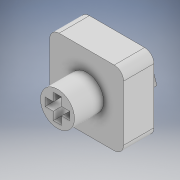
# Autodesk Inventor part: IPC A-CAL 9 key
Saved by Autodesk Inventor 2022 (Build 260153000, 153)
## iProperties
Created: 2021-12-31
Part Number: IPC A-CAL 9 key
Material: Generic
Document SubType Name: Modeling
Designer: solor
Density: 1 g/cm^3
Appearance: Default
Author: solor
Autodesk Inventor part; units mm, degrees
ref_plane "YZ Plane" through (0, 0, 0) normal (1, 0, 0) x (0, 1, 0)
ref_plane "XZ Plane" through (0, 0, 0) normal (0, 1, 0) x (-1, 0, 0)
sketch "Sketch1" plane through (0, 0, 0) normal (0, 0, 1) x (1, 0, 0)
  line L0 (14.6962, 12.74) -> (14.6962, 0) construction
  line L1 (10.61, 12.2) -> (1.53, 12.2)
  arc A0 (1.53, 12.2) -> (0, 10.67) centre (1.53, 10.67) ccw
  line L2 (0, 10.67) -> (0, 1.53)
  arc A1 (0, 1.53) -> (1.53, 0) centre (1.53, 1.53) ccw
  line L3 (1.53, 0) -> (10.61, 0)
  arc A2 (10.61, 0) -> (12.14, 1.53) centre (10.61, 1.53) ccw
  arc A3 (12.14, 10.67) -> (10.61, 12.2) centre (10.61, 10.67) ccw
  line L4 (12.14, 10.67) -> (12.14, 1.53)
  point P0 (0, 0)
  point P1 (0, 0)
  dimension "d10" = 12.74
  constraints: 10 end point, 8 point on circle, 4 centre point, 2 vertical, 1 point on line
  measures "d10" distance of L0.start L0.end
ref_plane "Work Plane1" through (0, 0, 5) normal (0, 0, 1) x (1, 0, 0)
sketch "Sketch2" plane through (0, 0, 5) normal (0, 0, 1) x (1, 0, 0)
  line L0 (10.88, 12.74) -> (1.8, 12.74) projected
  line L1 (10.88, 12.74) -> (1.8, 12.74) projected
  arc A0 (1.8, 12.74) -> (0, 10.94) centre (1.8, 10.94) ccw projected
  line L2 (0, 10.94) -> (0, 1.8) projected
  arc A1 (0, 1.8) -> (1.8, 0) centre (1.8, 1.8) ccw projected
  line L3 (1.8, 0) -> (10.88, 0) projected
  arc A2 (10.88, 0) -> (12.68, 1.8) centre (10.88, 1.8) ccw projected
  line L4 (12.68, 1.8) -> (12.68, 10.94) projected
  arc A3 (12.68, 10.94) -> (10.88, 12.74) centre (10.88, 10.94) ccw projected
  circle A4 centre (6.34, 6.37) radius 2.8
  line L5 (5.665, 8.395) -> (7.015, 8.395)
  line L6 (7.015, 4.345) -> (5.665, 4.345)
  line L7 (5.665, 4.345) -> (7.015, 8.395) construction
  line L8 (5.665, 8.395) -> (7.015, 4.345) construction
  line L9 (8.365, 5.695) -> (8.365, 7.045)
  line L10 (4.315, 7.045) -> (4.315, 5.695)
  line L11 (4.315, 5.695) -> (8.365, 7.045) construction
  line L12 (8.365, 5.695) -> (4.315, 7.045) construction
  line L13 (4.315, 5.695) -> (5.665, 5.695)
  line L14 (7.015, 5.695) -> (8.365, 5.695)
  line L15 (5.665, 4.345) -> (5.665, 5.695)
  line L16 (5.665, 7.045) -> (5.665, 8.395)
  line L17 (8.365, 7.045) -> (7.015, 7.045)
  line L18 (5.665, 7.045) -> (4.315, 7.045)
  line L19 (7.015, 8.395) -> (7.015, 7.045)
  line L20 (7.015, 5.695) -> (7.015, 4.345)
  point P0 (0, 0)
  dimension "d3" = 5.6
  dimension "d4" = 4.05
  dimension "d5" = 1.35
  dimension "d6" = 4.05
  dimension "d7" = 1.35
  constraints: 32 end point, 10 parallel, 8 perpendicular, 4 midpoint, 2 vertical, 1 centre point
  measures "d3" diameter of A4
  measures "d4" distance of L6.end L5.start
  measures "d5" distance of L5.start L5.end
  measures "d6" distance of L10.end L9.start
  measures "d7" distance of L9.end L9.start
extrude "Extrusion3" add sketch "Sketch1" along normal blind 5
sketch "Sketch3" plane through (0, 0, 5) normal (0, 0, 1) x (1, 0, 0)
  line L0 (10.61, 12.47) -> (1.53, 12.47)
  line L1 (10.61, 12.47) -> (1.53, 12.47)
  arc A0 (1.53, 12.47) -> (-0.27, 10.67) centre (1.53, 10.67) ccw
  line L2 (-0.27, 10.67) -> (-0.27, 1.53)
  arc A1 (-0.27, 1.53) -> (1.53, -0.27) centre (1.53, 1.53) ccw
  line L3 (1.53, -0.27) -> (10.61, -0.27)
  arc A2 (10.61, -0.27) -> (12.41, 1.53) centre (10.61, 1.53) ccw
  line L4 (12.41, 1.53) -> (12.41, 10.67)
  arc A3 (12.41, 10.67) -> (10.61, 12.47) centre (10.61, 10.67) ccw
  circle A4 centre (6.07, 6.1) radius 2.8
  line L5 (5.395, 8.125) -> (6.745, 8.125)
  line L6 (6.745, 4.075) -> (5.395, 4.075)
  line L7 (5.395, 4.075) -> (6.745, 8.125) construction
  line L8 (5.395, 8.125) -> (6.745, 4.075) construction
  line L9 (8.095, 5.425) -> (8.095, 6.775)
  line L10 (4.045, 6.775) -> (4.045, 5.425)
  line L11 (4.045, 5.425) -> (8.095, 6.775) construction
  line L12 (8.095, 5.425) -> (4.045, 6.775) construction
  line L13 (4.045, 5.425) -> (5.395, 5.425)
  line L14 (6.745, 5.425) -> (8.095, 5.425)
  line L15 (5.395, 4.075) -> (5.395, 5.425)
  line L16 (5.395, 6.775) -> (5.395, 8.125)
  line L17 (8.095, 6.775) -> (6.745, 6.775)
  line L18 (5.395, 6.775) -> (4.045, 6.775)
  line L19 (6.745, 8.125) -> (6.745, 6.775)
  line L20 (6.745, 5.425) -> (6.745, 4.075)
  line L21 (10.61, 12.2) -> (1.53, 12.2) projected
  line L22 (0, 10.67) -> (0, 1.53) projected
  point P0 (0, 0)
  point P1 (-0.27, -0.27)
  point P2 (6.07, 12.2)
  point P3 (0, 6.1)
  point P4 (6.07, 6.1)
  dimension "d14" = 5.6
  dimension "d15" = 4.05
  dimension "d16" = 1.35
  dimension "d17" = 4.05
  dimension "d18" = 1.35
  constraints: 42 end point, 10 parallel, 8 perpendicular, 8 point on circle, 6 midpoint, 5 centre point, 2 vertical
  measures "d14" diameter of A4
  measures "d15" distance of L6.end L5.start
  measures "d16" distance of L5.start L5.end
  measures "d17" distance of L10.end L9.start
  measures "d18" distance of L9.end L9.start
extrude "Extrusion4" add sketch "Sketch3" along normal blind 4.8 contours A4
sketch "Sketch4" plane through (0, 0, 0) normal (0, 0, -1) x (-1, 0, 0)
  line L0 (-13.9436, 0) -> (-13.9436, 2.266)
  line L1 (-15.5559, 0) -> (-15.5559, 6.84)
  line L2 (-1.53, 0) -> (-10.61, 0) projected
  line L3 (-11.7151, 9.645) -> (-0.4249, 9.645) construction
  line L4 (-0.4249, 9.645) -> (-0.4249, 6.84) construction
  line L5 (-0.4249, 6.84) -> (-11.7151, 6.84) construction
  line L6 (-11.7151, 6.84) -> (-11.7151, 9.645) construction
  line L7 (-7.4059, 5.4371) -> (-4.7341, 5.4371) construction
  line L8 (-4.7341, 5.4371) -> (-4.7341, 2.266) construction
  line L9 (-4.7341, 2.266) -> (-7.4059, 2.266) construction
  line L10 (-7.4059, 2.266) -> (-7.4059, 5.4371) construction
  line L11 (-11.726, 6.8925) -> (-10.8136, 9.5925)
  line L12 (-10.8136, 9.5925) -> (-10.0741, 9.5925)
  line L13 (-10.0741, 9.5925) -> (-9.1617, 6.8925)
  line L14 (-9.1617, 6.8925) -> (-9.8596, 6.8925)
  line L15 (-9.8596, 6.8925) -> (-10.0281, 7.4439)
  line L16 (-10.0281, 7.4439) -> (-10.8771, 7.4439)
  line L17 (-10.8771, 7.4439) -> (-11.0477, 6.8925)
  line L18 (-11.0477, 6.8925) -> (-11.726, 6.8925)
  line L19 (-10.1769, 7.934) -> (-10.4526, 8.8267)
  line L20 (-10.4526, 8.8267) -> (-10.7305, 7.934)
  line L21 (-10.7305, 7.934) -> (-10.1769, 7.934)
  line L22 (-7.7723, 7.8334) -> (-8.9735, 7.8334)
  line L23 (-8.9735, 7.8334) -> (-8.9735, 8.3366)
  line L24 (-8.9735, 8.3366) -> (-7.7723, 8.3366)
  line L25 (-7.7723, 8.3366) -> (-7.7723, 7.8334)
  spline S0 degree 2 poles (-6.1269, 6.84) (-6.7352, 6.84) (-7.4484, 7.5752) (-7.4484, 8.2403) knots 0 0 0 1 2 2 2
  spline S1 degree 2 poles (-7.4484, 8.2403) (-7.4484, 8.8814) (-6.733, 9.645) (-6.1247, 9.645) knots 0 0 0 1 2 2 2
  spline S2 degree 2 poles (-6.1247, 9.645) (-5.965, 9.645) (-5.7068, 9.6078) (-5.5886, 9.5772) knots 0 0 0 1 2 2 2
  spline S3 degree 2 poles (-5.5886, 9.5772) (-5.4967, 9.5488) (-5.2801, 9.4547) (-5.2123, 9.4197) knots 0 0 0 1 2 2 2
  line L26 (-5.2123, 9.4197) -> (-5.2123, 8.7764)
  line L27 (-5.2123, 8.7764) -> (-5.2801, 8.7764)
  spline S4 degree 2 poles (-5.2801, 8.7764) (-5.3305, 8.8201) (-5.4792, 8.9427) (-5.5733, 8.9996) knots 0 0 0 1 2 2 2
  spline S5 degree 2 poles (-5.5733, 8.9996) (-5.6674, 9.0586) (-5.8928, 9.1396) (-6.0175, 9.1396) knots 0 0 0 1 2 2 2
  spline S6 degree 2 poles (-6.0175, 9.1396) (-6.1641, 9.1396) (-6.407, 9.0477) (-6.5185, 8.9317) knots 0 0 0 1 2 2 2
  spline S7 degree 2 poles (-6.5185, 8.9317) (-6.6192, 8.8289) (-6.7483, 8.4766) (-6.7483, 8.2381) knots 0 0 0 1 2 2 2
  spline S8 degree 2 poles (-6.7483, 8.2381) (-6.7483, 7.9865) (-6.6148, 7.643) (-6.5054, 7.538) knots 0 0 0 1 2 2 2
  spline S9 degree 2 poles (-6.5054, 7.538) (-6.4004, 7.4351) (-6.1422, 7.3454) (-6.0131, 7.3454) knots 0 0 0 1 2 2 2
  spline S10 degree 2 poles (-6.0131, 7.3454) (-5.8796, 7.3454) (-5.6368, 7.4351) (-5.5536, 7.4898) knots 0 0 0 1 2 2 2
  spline S11 degree 2 poles (-5.5536, 7.4898) (-5.4617, 7.5445) (-5.3239, 7.6605) (-5.2736, 7.7065) knots 0 0 0 1 2 2 2
  line L28 (-5.2736, 7.7065) -> (-5.2123, 7.7065)
  line L29 (-5.2123, 7.7065) -> (-5.2123, 7.0719)
  spline S12 degree 2 poles (-5.2123, 7.0719) (-5.2867, 7.0369) (-5.4814, 6.9494) (-5.5865, 6.9188) knots 0 0 0 1 2 2 2
  spline S13 degree 2 poles (-5.5865, 6.9188) (-5.7134, 6.8794) (-5.9343, 6.84) (-6.1269, 6.84) knots 0 0 0 1 2 2 2
  line L30 (-5.1029, 6.8925) -> (-4.1905, 9.5925)
  line L31 (-4.1905, 9.5925) -> (-3.451, 9.5925)
  line L32 (-3.451, 9.5925) -> (-2.5386, 6.8925)
  line L33 (-2.5386, 6.8925) -> (-3.2365, 6.8925)
  line L34 (-3.2365, 6.8925) -> (-3.405, 7.4439)
  line L35 (-3.405, 7.4439) -> (-4.254, 7.4439)
  line L36 (-4.254, 7.4439) -> (-4.4246, 6.8925)
  line L37 (-4.4246, 6.8925) -> (-5.1029, 6.8925)
  line L38 (-3.5538, 7.934) -> (-3.8295, 8.8267)
  line L39 (-3.8295, 8.8267) -> (-4.1074, 7.934)
  line L40 (-4.1074, 7.934) -> (-3.5538, 7.934)
  line L41 (-0.4687, 6.8925) -> (-2.2694, 6.8925)
  line L42 (-2.2694, 6.8925) -> (-2.2694, 9.5925)
  line L43 (-2.2694, 9.5925) -> (-1.5912, 9.5925)
  line L44 (-1.5912, 9.5925) -> (-1.5912, 7.4067)
  line L45 (-1.5912, 7.4067) -> (-0.4687, 7.4067)
  line L46 (-0.4687, 7.4067) -> (-0.4687, 6.8925)
  spline S14 degree 2 poles (-4.9343, 4.0209) (-4.9343, 3.6328) (-5.1147, 2.9852) (-5.305, 2.7529) knots 0 0 0 1 2 2 2
  spline S15 degree 2 poles (-5.305, 2.7529) (-5.5028, 2.5181) (-6.0861, 2.266) (-6.5112, 2.266) knots 0 0 0 1 2 2 2
  spline S16 degree 2 poles (-6.5112, 2.266) (-6.6545, 2.266) (-6.966, 2.3031) (-7.0179, 2.3179) knots 0 0 0 1 2 2 2
  line L47 (-7.0179, 2.3179) -> (-7.0179, 2.916)
  line L48 (-7.0179, 2.916) -> (-6.9586, 2.916)
  spline S17 degree 2 poles (-6.9586, 2.916) (-6.9017, 2.8864) (-6.6891, 2.8221) (-6.5038, 2.8221) knots 0 0 0 1 2 2 2
  spline S18 degree 2 poles (-6.5038, 2.8221) (-6.353, 2.8221) (-6.0737, 2.9012) (-5.9748, 2.9877) knots 0 0 0 1 2 2 2
  spline S19 degree 2 poles (-5.9748, 2.9877) (-5.8686, 3.0792) (-5.7301, 3.3486) (-5.7054, 3.5513) knots 0 0 0 1 2 2 2
  spline S20 degree 2 poles (-5.7054, 3.5513) (-5.8686, 3.4499) (-6.1503, 3.3412) (-6.3604, 3.3412) knots 0 0 0 1 2 2 2
  spline S21 degree 2 poles (-6.3604, 3.3412) (-6.5161, 3.3412) (-6.8053, 3.4252) (-6.924, 3.5142) knots 0 0 0 1 2 2 2
  spline S22 degree 2 poles (-6.924, 3.5142) (-7.0821, 3.6353) (-7.2675, 4.0233) (-7.2675, 4.3298) knots 0 0 0 1 2 2 2
  spline S23 degree 2 poles (-7.2675, 4.3298) (-7.2675, 4.5696) (-7.1044, 4.9724) (-6.9561, 5.1207) knots 0 0 0 1 2 2 2
  spline S24 degree 2 poles (-6.9561, 5.1207) (-6.8078, 5.269) (-6.3777, 5.4371) (-6.1133, 5.4371) knots 0 0 0 1 2 2 2
  spline S25 degree 2 poles (-6.1133, 5.4371) (-5.8463, 5.4371) (-5.4336, 5.2888) (-5.2853, 5.1331) knots 0 0 0 1 2 2 2
  spline S26 degree 2 poles (-5.2853, 5.1331) (-5.1122, 4.9601) (-4.9343, 4.4114) (-4.9343, 4.0209) knots 0 0 0 1 2 2 2
  spline S27 degree 2 poles (-5.6931, 4.1346) (-5.6931, 4.3842) (-5.7771, 4.7055) (-5.8537, 4.7945) knots 0 0 0 1 2 2 2
  spline S28 degree 2 poles (-5.8537, 4.7945) (-5.9056, 4.8612) (-6.0391, 4.9181) (-6.1157, 4.9181) knots 0 0 0 1 2 2 2
  spline S29 degree 2 poles (-6.1157, 4.9181) (-6.1849, 4.9181) (-6.3135, 4.8637) (-6.3728, 4.7945) knots 0 0 0 1 2 2 2
  spline S30 degree 2 poles (-6.3728, 4.7945) (-6.4247, 4.7352) (-6.4988, 4.5053) (-6.4988, 4.3694) knots 0 0 0 1 2 2 2
  spline S31 degree 2 poles (-6.4988, 4.3694) (-6.4988, 4.2211) (-6.4222, 4.0307) (-6.3579, 3.9739) knots 0 0 0 1 2 2 2
  spline S32 degree 2 poles (-6.3579, 3.9739) (-6.2912, 3.9171) (-6.1256, 3.8726) (-6.0218, 3.8726) knots 0 0 0 1 2 2 2
  spline S33 degree 2 poles (-6.0218, 3.8726) (-5.9353, 3.8726) (-5.7549, 3.9195) (-5.698, 3.9442) knots 0 0 0 1 2 2 2
  spline S34 degree 2 poles (-5.698, 3.9442) (-5.698, 3.9665) (-5.6931, 4.0505) (-5.6931, 4.1346) knots 0 0 0 1 2 2 2
  point P0 (0, 0)
  point P1 (-6.07, 0)
  point P2 (-6.07, 2.266)
  point P3 (-6.07, 6.84)
  point P4 (-6.07, 6.84)
  point P5 (-6.07, 2.266)
  dimension "d21" = 2.266
  dimension "d22" = 6.84
  constraints: 4 end point, 3 midpoint, 2 vertical, 4 other
  measures "d21" distance of L0.start L0.end
  measures "d22" distance of L1.start L1.end
extrude "Extrusion5" add sketch "Sketch4" along normal blind 0.9
body "Solid2"
